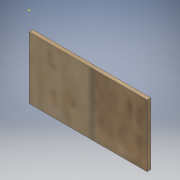
# Autodesk Inventor part: inferior y superior
Saved by Autodesk Inventor 2018 (Build 220112000, 112)
## iProperties
Created: 2019-02-27
Part Number: inferior y superior
Material: Madera (arce)
Document SubType Name: Modeling
Designer: USUARIO WINDOWS
Density: 0.67 g/cm^3
Appearance: Arce natural - De color oscuro brillante
Author: USUARIO WINDOWS
Autodesk Inventor part; units mm, degrees
ref_plane "YZ Plane" through (0, 0, 0) normal (1, 0, 0) x (0, 1, 0)
ref_plane "XZ Plane" through (0, 0, 0) normal (0, 1, 0) x (-1, 0, 0)
ref_plane "XY Plane" through (0, 0, 0) normal (0, 0, 1) x (1, 0, 0)
sketch "Boceto1" plane through (0, 0, 0) normal (0, 1, 0) x (-1, 0, 0)
  point P0 (0, 0)
sketch "Boceto2" plane through (0, 0, 0) normal (0, 1, 0) x (-1, 0, 0)
  line L0 (0, 0) -> (-105, 0)
  line L1 (-105, 0) -> (-105, -70)
  line L2 (-105, -70) -> (0, -70)
  line L3 (0, -70) -> (0, 0)
  dimension "d0" = 105
  dimension "d1" = 70
  constraints: 8 end point, 2 parallel, 1 horizontal, 1 perpendicular
  measures "d0" distance of L2.end L1.end
  measures "d1" distance of L1.end L0.end
extrude "Extrusión1" add sketch "Boceto2" along normal blind 3
sketch "Boceto3" plane through (0, 0, 0) normal (0, -1, 0) x (1, 0, 0)
  point P0 (0, 0)
sketch "Boceto4" plane through (105, 0, 0) normal (1, 0, 0) x (0, 0, -1)
  line L0 (0, 0) -> (70, 0) projected
  line L1 (70, 0) -> (70, 3) projected
  line L2 (0, 3) -> (70, 3) projected
  line L3 (0, 0) -> (0, 3) projected
extrude "Extrusión2" cut sketch "Boceto4" against normal blind 5
sketch "Boceto5" plane through (100, 0, 0) normal (1, 0, 0) x (0, 0, -1)
  line L0 (0, 3) -> (70, 3) projected
  line L1 (70, 0) -> (0, 0) projected
  line L2 (70, 3) -> (70, 0) projected
  line L3 (0, 3) -> (70, 3) projected
  line L4 (0, 0) -> (0, 3) projected
extrude "Extrusión3" cut sketch "Boceto5" against normal blind 5
sketch "Boceto6" plane through (0, 0, 0) normal (0, -1, 0) x (1, 0, 0)
  line L0 (95, -70) -> (95, 0) projected
  line L1 (0, 0) -> (95, 0) projected
  line L2 (0, -70) -> (0, 0) projected
  line L3 (95, -70) -> (0, -70) projected
  line L4 (0, -70) -> (0, 0) projected
  line L5 (0, 0) -> (90, 0)
  line L6 (90, 0) -> (90, -65)
  line L7 (90, -65) -> (0, -65)
  line L8 (0, -65) -> (0, 0)
  dimension "d8" = 90
  dimension "d9" = 65
  constraints: 8 end point, 2 parallel, 1 horizontal, 1 perpendicular
  measures "d8" distance of L6.end L7.end
  measures "d9" distance of L5.end L6.end
extrude "Extrusión4" cut sketch "Boceto6" against normal blind 5 contours L3 L2 L7 L6 L1 L0
sketch "Boceto7" plane through (90, 0, 0) normal (1, 0, 0) x (0, 0, -1)
  line L0 (0, 3) -> (65, 3) projected
  line L1 (0, 0) -> (0, 3) projected
  line L2 (65, 0) -> (0, 0) projected
  line L3 (65, 0) -> (65, 3) projected
extrude "Extrusión5" add sketch "Boceto7" along normal blind 5
sketch "Boceto8" plane through (0, 0, 0) normal (0, 0, 1) x (1, 0, 0)
  line L0 (0, 3) -> (95, 3) projected
  line L1 (0, 0) -> (0, 3) projected
  line L2 (0, 0) -> (95, 0) projected
  line L3 (95, 3) -> (95, 0) projected
extrude "Extrusión6" cut sketch "Boceto8" against normal blind 15
